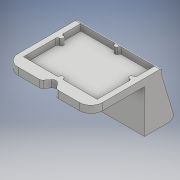
# Autodesk Inventor part: TUBE_PCB
Saved by Autodesk Inventor 2018 (Build 220112000, 112)
## iProperties
Created: 2020-08-08
Part Number: TUBE_PCB
Material: Generic
Document SubType Name: Modeling
Designer: sawer
Density: 1 g/cm^3
Appearance: Default
Author: sawer
Autodesk Inventor part; units mm, degrees
ref_plane "YZ Plane" through (0, 0, 0) normal (1, 0, 0) x (0, 1, 0)
ref_plane "XZ Plane" through (0, 0, 0) normal (0, 1, 0) x (-1, 0, 0)
ref_plane "XY Plane" through (0, 0, 0) normal (0, 0, 1) x (1, 0, 0)
sketch "Sketch1" plane through (0, 0, 0) normal (0, 0, 1) x (1, 0, 0)
  line L0 (0, 0) -> (10.9, 0) construction
  line L1 (10.9, 0) -> (10.9, 9.15)
  line L2 (10.9, 9.15) -> (-10.9, 9.15)
  line L3 (-10.9, 9.15) -> (-10.9, -6.15)
  line L4 (10.9, -6.15) -> (10.9, 0)
  line L5 (0, -9.15) -> (0, -5.65) construction
  arc A0 (7.9, -9.15) -> (10.9, -6.15) centre (7.9, -6.15) ccw
  arc A1 (-10.9, -6.15) -> (-7.9, -9.15) centre (-7.9, -6.15) ccw
  line L6 (0, -9.15) -> (2, -9.15) construction
  line L7 (0, -9.15) -> (0, -6.65) construction
  line L8 (0, -6.65) -> (2, -9.15)
  line L9 (-2, -9.15) -> (0, -6.65)
  line L10 (-7.9, -9.15) -> (-2, -9.15)
  line L11 (2, -9.15) -> (7.9, -9.15)
  point P0 (-10.9, -9.15)
  point P1 (10.9, -9.15)
  dimension "d0" = 10.9
  dimension "d1" = 9.15
  dimension "d2" = 21.8
  dimension "d3" = 18.3
  dimension "d4" = 21.8
  dimension "d6" = 3
  constraints: 24 end point, 6 tangent, 4 point on circle, 4 point on line, 2 centre point, 2 perpendicular, 2 vertical, 1 equal radius, 1 horizontal
  measures "d0" distance of L0.start L0.end
  measures "d1" distance of L0.end L1.end
  measures "d2" distance of L1.end L2.end
  measures "d3" distance of L2.end point (-10.9, -9.15)
  measures "d4" distance of point (-10.9, -9.15) point (10.9, -9.15)
  measures "d6" radius of A0
extrude "Extrusion1" add sketch "Sketch1" along normal blind 1.85
fillet "Fillet2" radius 1 3 edges at (0, -6.65, 0.925) (-2, -9.15, 0.925) (2, -9.15, 0.925)
sketch "Sketch5" plane through (0, 0, 1.85) normal (0, 0, 1) x (1, 0, 0)
  line L0 (10.9, -6.15) -> (10.9, 9.15) construction
  line L1 (10.9, -6.15) -> (9.5, -6.15) construction
  line L2 (10.9, 9.15) -> (10.9, 8.65) construction
  line L3 (10.9, 8.65) -> (9.5, 8.65) construction
  line L4 (-9.5, 8.65) -> (-9.5, 3.65) construction
  line L5 (-9.5, 3.65) -> (-9, 3.65)
  line L6 (-8.5, 3.15) -> (-8.5, 3.15)
  line L7 (-9, 2.65) -> (-9.5, 2.65)
  line L8 (9.5, 8.65) -> (9.5, 3.65) construction
  line L9 (9.5, 3.65) -> (9, 3.65)
  line L10 (8.5, 3.15) -> (8.5, 3.15)
  line L11 (9, 2.65) -> (9.5, 2.65)
  arc A0 (8.5, 3.15) -> (9, 2.65) centre (9, 3.15) ccw
  arc A1 (9, 3.65) -> (8.5, 3.15) centre (9, 3.15) ccw
  arc A2 (-9, 2.65) -> (-8.5, 3.15) centre (-9, 3.15) ccw
  arc A3 (-8.5, 3.15) -> (-9, 3.65) centre (-9, 3.15) ccw
  line L12 (0, 8.65) -> (0.5, 8.65) construction
  line L13 (0.5, 8.65) -> (0.5, 8.275)
  line L14 (0.125, 7.9) -> (-0.125, 7.9)
  line L15 (-0.5, 8.275) -> (-0.5, 8.65)
  line L16 (0, -6.15) -> (0.5, -6.15) construction
  line L17 (0.5, -6.15) -> (0.5, -5.775)
  line L18 (0.125, -5.4) -> (-0.125, -5.4)
  line L19 (-0.5, -5.775) -> (-0.5, -6.15)
  arc A4 (0.5, -5.775) -> (0.125, -5.4) centre (0.125, -5.775) ccw
  arc A5 (-0.125, -5.4) -> (-0.5, -5.775) centre (-0.125, -5.775) ccw
  arc A6 (-0.5, 8.275) -> (-0.125, 7.9) centre (-0.125, 8.275) ccw
  arc A7 (0.125, 7.9) -> (0.5, 8.275) centre (0.125, 8.275) ccw
  line L20 (9.5, 8.65) -> (0.5, 8.65)
  line L21 (-0.5, 8.65) -> (-9.5, 8.65)
  line L22 (-9.5, 8.65) -> (-9.5, 3.65)
  line L23 (-9.5, 2.65) -> (-9.5, -6.15)
  line L24 (9.5, -6.15) -> (0.5, -6.15)
  line L25 (-0.5, -6.15) -> (-9.5, -6.15)
  line L26 (9.5, -6.15) -> (9.5, 2.65)
  line L27 (9.5, 3.65) -> (9.5, 8.65)
  point P0 (0, 0)
  point P1 (-8.5, 3.65)
  point P2 (-8.5, 2.65)
  point P3 (8.5, 3.65)
  point P4 (8.5, 2.65)
  point P5 (0.5, 7.9)
  point P6 (-0.5, 7.9)
  point P7 (0.5, -5.4)
  point P8 (-0.5, -5.4)
  dimension "d33" = 1.4
  dimension "d34" = 0.5
  dimension "d35" = 1.4
  dimension "d77" = 19
  dimension "d78" = 5
  dimension "d79" = 1
  dimension "d80" = 1
  dimension "d81" = 5
  dimension "d82" = 1
  dimension "d83" = 1
  dimension "d84" = 0.5
  dimension "d85" = 0.5
  dimension "d86" = 0.75
  dimension "d87" = 1
  dimension "d88" = 0.5
  dimension "d89" = 0.75
  dimension "d90" = 1
  dimension "d91" = 0.375
  constraints: 54 end point, 17 point on line, 16 point on circle, 16 tangent, 15 perpendicular, 8 centre point, 6 equal radius, 5 horizontal, 3 vertical
  measures "d33" distance of L0.start L1.end
  measures "d34" distance of L0.end L2.end
  measures "d35" distance of L2.end L3.end
  measures "d77" distance of L3.end L4.start
  measures "d78" distance of L4.start L4.end
  measures "d79" distance of L4.end point (-8.5, 3.65)
  measures "d80" distance of point (-8.5, 3.65) point (-8.5, 2.65)
  measures "d81" distance of L3.end L8.end
  measures "d82" distance of L8.end point (8.5, 3.65)
  measures "d83" distance of point (8.5, 3.65) point (8.5, 2.65)
  measures "d84" radius of A0
  measures "d85" distance of L12.start L12.end
  measures "d86" distance of L12.end point (0.5, 7.9)
  measures "d87" distance of point (0.5, 7.9) point (-0.5, 7.9)
  measures "d88" distance of L16.start L16.end
  measures "d89" distance of L16.end point (0.5, -5.4)
  measures "d90" distance of point (0.5, -5.4) point (-0.5, -5.4)
  measures "d91" radius of A4
extrude "Extrusion4" cut sketch "Sketch5" against normal blind 1.65
sketch "Sketch6" plane through (-10.9, 9.15, 0) normal (0, 1, 0) x (1, 0, 0)
  line L0 (0, 0) -> (0, -1.85) construction
  line L1 (21.8, 0) -> (21.8, -1.85) construction
  line L2 (0, 0) -> (21.8, 0) construction
  line L3 (10.9, 0) -> (10.9, -1.85) construction
  line L4 (10.9, -1.85) -> (10.9, 11.15) construction
  line L5 (10.9, 11.15) -> (0, 11.15)
  line L6 (0, 11.15) -> (0, 0)
  line L7 (21.8, 0) -> (21.8, 11.15)
  line L8 (0, 11.15) -> (21.8, 11.15)
  line L9 (0, 0) -> (21.8, 0)
  dimension "d40" = 13
  dimension "d41" = 10.9
  dimension "d42" = 10.9
  constraints: 16 end point, 4 horizontal, 2 vertical
  measures "d40" distance of L3.end L4.end
  measures "d41" distance of L4.end L7.end
  measures "d42" distance of L4.end L5.end
extrude "Extrusion5" add sketch "Sketch6" against normal blind 4.5
fillet "Fillet3" radius 0.5 1 edges at (0, 9.15, 1.85)
sketch "Sketch7" plane through (-10.9, 9.15, -11.15) normal (0, 1, 0) x (1, 0, 0)
  line L0 (0, -11.15) -> (0, -13) projected
  line L1 (0, -11.15) -> (1.5, -11.15)
  line L2 (1.5, -11.15) -> (1.5, 0)
  line L3 (0, 0) -> (21.8, 0) projected
  line L4 (0, 0) -> (0, -11.15)
  line L5 (0, -11.15) -> (1.5, -11.15)
  line L6 (21.8, -11.15) -> (20.3, -11.15)
  line L7 (20.3, -11.15) -> (20.3, 0)
  line L8 (21.8, 0) -> (21.8, -11.15)
  line L9 (21.8, 0) -> (21.8, -12.5) projected
  point P0 (10.9, -11.15)
  dimension "d46" = 1.5
  dimension "d53" = 1.5
  constraints: 14 end point, 3 horizontal, 2 perpendicular, 2 point on line, 1 collinear, 1 parallel
  measures "d46" distance of L0.start L1.end
  measures "d53" distance of L6.start L6.end
extrude "Extrusion6" add sketch "Sketch7" along normal blind 3
chamfer "Chamfer1" distance 10 distance2 3 1 edges at (-10.15, 12.15, 0) measured on face at (-10.15, 12.15, -0.5)
fillet "Fillet4" radius 1.25 1 edges at (-10.15, 12.15, -11.15)
chamfer "Chamfer2" distance 10 distance2 3 1 edges at (10.15, 12.15, 0) measured on face at (10.15, 12.15, -0.5)
fillet "Fillet5" radius 1.25 1 edges at (10.15, 12.15, -11.15)
fillet "Fillet7" radius 0.5 8 edges at (-0.5, 8.65, 1.025) (9.5, 2.65, 1.025) (-9.5, 3.65, 1.025) (0.5, -6.15, 1.025) (9.5, 3.65, 1.025) (-0.5, -6.15, 1.025) (0.5, 8.65, 1.025) (-9.5, 2.65, 1.025)
body "Solid1"
